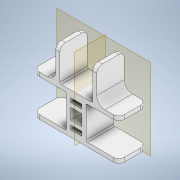
# Autodesk Inventor part: fuselage_tail_interface_airfoiled
Saved by Autodesk Inventor 2021 (Build 250183000, 183)
## iProperties
Created: 2020-11-20
Part Number: fuselage_tail_interface_airfoiled
Material: ABS Plastic
Document SubType Name: Modeling
Designer: Paco
Density: 1.06 g/cm^3
Appearance: Smooth - White
Mass: 1.99311 g
Surface Area: 25.7447 cm^2
Volume: 1.8803 cm^3
Author: Paco
Autodesk Inventor part; units mm, degrees
ref_plane "XZ Plane" through (0, 0, 0) normal (0, 1, 0) x (-1, 0, 0)
sketch "Sketch1" plane through (0, 0, 0) normal (0, 0, 1) x (1, 0, 0)
  line L0 (-2.05, 2.05) -> (2.05, 2.05)
  line L1 (2.05, 2.05) -> (2.05, -2.05)
  line L2 (2.05, -2.05) -> (-2.05, -2.05)
  line L3 (-2.05, -2.05) -> (-2.05, 2.05)
  line L4 (0, 2.05) -> (0, -2.05) construction
  line L5 (0, 7.5) -> (-15.55, 7.5)
  line L6 (-15.55, 7.5) -> (-15.55, 6)
  line L7 (-15.55, 6) -> (-3.55, 6)
  line L8 (-3.55, 6) -> (-3.55, -6)
  line L9 (-3.55, -6) -> (-15.55, -6)
  line L10 (-15.55, -6) -> (-15.55, -7.5)
  line L11 (-15.55, -7.5) -> (-0.55, -7.5)
  line L12 (-2.05, 0) -> (2.05, 0) construction
  line L13 (0, 7.5) -> (15.55, 7.5)
  line L14 (15.55, 7.5) -> (15.55, 6)
  line L15 (15.55, 6) -> (3.55, 6)
  line L16 (3.55, 6) -> (3.55, -6)
  line L17 (3.55, -6) -> (15.55, -6)
  line L18 (15.55, -6) -> (15.55, -7.5)
  line L19 (15.55, -7.5) -> (-0.55, -7.5)
  line L20 (-2.05, 2.05) -> (2.05, -2.05) construction
  line L21 (2.05, 2.05) -> (-2.05, -2.05) construction
  line L22 (0, 7.5) -> (0, 2.05) construction
  point P0 (0, 0)
  point P1 (0, 0)
  point P2 (0, 0)
  dimension "d3" = 4.1
  dimension "d4" = 4.1
  dimension "d5" = 12
  dimension "d6" = 1.5
  dimension "d7" = 1.5
  dimension "d8" = 5.45
  dimension "d9" = 5.45
  dimension "d10" = 1.5
  dimension "d11" = 12
  dimension "d37" = 15
  constraints: 46 end point, 7 perpendicular, 6 midpoint, 6 symmetric about line, 4 point on line, 2 horizontal, 2 parallel, 1 coincident, 1 other
  measures "d3" distance of L0.start L0.end
  measures "d4" distance of L0.end L1.end
  measures "d5" distance between parallel lines of L9 L7
  measures "d6" distance of L5.end L6.end
  measures "d7" distance of L9.end L10.end
  measures "d8" distance between parallel lines of L0 L5
  measures "d9" distance between parallel lines of L11 L2
  measures "d10" distance between parallel lines of L8 L3
  measures "d11" distance of L6.end L7.end
  measures "d37" distance between parallel lines of L11 L5
extrude "Extrusion1" add sketch "Sketch1" along normal blind 10
sketch "Sketch5" plane through (0, 0, 10) normal (0, 0, 1) x (1, 0, 0)
  line L0 (6, 19.5) -> (7.5, 19.5)
  line L1 (7.5, 19.5) -> (7.5, 7.5)
  line L2 (7.5, 7.5) -> (6, 7.5)
  line L3 (6, 7.5) -> (6, 19.5)
  line L4 (15.55, 7.5) -> (-15.55, 7.5) projected
  line L5 (3.55, -6) -> (3.55, 6) projected
  line L6 (0, 0) -> (0, 23.4065) construction
  dimension "d41" = 1.5
  dimension "d42" = 12
  dimension "d47" = 6
  constraints: 10 end point, 2 parallel, 2 vertical, 1 collinear, 1 horizontal, 1 perpendicular
  measures "d41" distance of L0.start L0.end
  measures "d42" distance of L0.end L1.end
  measures "d47" distance between parallel lines of L3 L6
extrude "Extrusion5" add sketch "Sketch5" against normal up to surface (10 mm away)
mirror "Mirror1" about plane through (0, 0, 0) normal (1, 0, 0) of "Extrusion5"
fillet "Fillet1" radius 3 2 edges at (-7.5, 7.5, 5) (7.5, 7.5, 5)
fillet "Fillet2" radius 0.5 6 edges at (-3.55, 6, 5) (-3.55, -6, 5) (3.55, -6, 5) (3.55, 6, 5) (-6, 7.5, 5) (6, 7.5, 5)
fillet "Fillet3" radius 2 12 edges at (-6.75, 19.5, 10) (-15.55, 6.75, 10) (-6.75, 19.5, 0) (6.75, 19.5, 0) (6.75, 19.5, 10) (15.55, 6.75, 10) (15.55, 6.75, 0) (15.55, -6.75, 0) (15.55, -6.75, 10) (-15.55, -6.75, 10) (-15.55, -6.75, 0) (-15.55, 6.75, 0)
sketch "Sketch7" plane through (0, 0, 0) normal (0, 0, -1) x (-1, 0, 0)
  line L0 (-2.05, 5.05) -> (2.05, 5.05)
  line L1 (2.05, 5.05) -> (2.05, 3.55)
  line L2 (2.05, 3.55) -> (-2.05, 3.55)
  line L3 (-2.05, 3.55) -> (-2.05, 5.05)
  line L4 (-2.05, -3.55) -> (2.05, -3.55)
  line L5 (2.05, -3.55) -> (2.05, -5.05)
  line L6 (2.05, -5.05) -> (-2.05, -5.05)
  line L7 (-2.05, -5.05) -> (-2.05, -3.55)
  line L8 (2.05, 2.05) -> (-2.05, 2.05) projected
  line L9 (-2.05, -2.05) -> (2.05, -2.05) projected
  line L10 (2.05, -2.05) -> (2.05, 2.05) projected
  line L11 (-2.05, 2.05) -> (-2.05, -2.05) projected
  point P0 (0, 0)
  dimension "d55" = 1.5
  dimension "d56" = 1.5
  dimension "d57" = 1.5
  dimension "d58" = 1.5
  constraints: 16 end point, 4 parallel, 3 collinear, 2 horizontal, 2 perpendicular, 1 point on line
  measures "d55" distance of L0.end L1.end
  measures "d56" distance of L4.end L5.end
  measures "d57" distance between parallel lines of L8 L2
  measures "d58" distance between parallel lines of L4 L9
extrude "Extrusion7" cut sketch "Sketch7" against normal blind 10 contours L0 L1 L2 L3 | L4 L5 L6 L7
equation "\"d7\" = d6"
equation "\"d8\" = d9"
body "Solid1"
